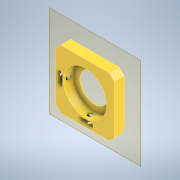
# Autodesk Inventor part: 20_Cube_Insert_Kinematic_KES400AMount_45_UPD_v3
Saved by Autodesk Inventor 2022 (Build 260153000, 153)
## iProperties
Created: 2021-11-15
Part Number: 20_Cube_Insert_Kinematic_KES400AMount_45_UPD_v3
Material: Generic
Document SubType Name: Modeling
Designer: diederichbenedict
Density: 1 g/cm^3
Appearance: Glossy - Gold
Author: diederichbenedict
Autodesk Inventor part; units mm, degrees
ref_plane "YZ Plane" through (0, 0, 0) normal (1, 0, 0) x (0, 1, 0)
ref_plane "XZ Plane" through (0, 0, 0) normal (0, 1, 0) x (-1, 0, 0)
ref_plane "XY Plane" through (0, 0, 0) normal (0, 0, 1) x (1, 0, 0)
ref_plane "Work Plane1" through (0, 0, 2) normal (0, 0, 1) x (1, 0, 0)
sketch "Sketch1" plane through (0, 0, 2) normal (0, 0, 1) x (1, 0, 0)
  circle A0 centre (-37.0712, 14) radius 3.25 construction
  circle A1 centre (-9.0712, -14) radius 3.25 construction
  line L0 (-21.8762, -24.9) -> (-21.8762, -17.08) construction
  line L1 (-21.8762, -17.08) -> (-20.0712, -17.08) construction
  arc A2 (-20.0712, -17.08) -> (-20.0712, -14.08) centre (-20.0712, -15.58) ccw construction
  line L2 (-20.0712, -14.08) -> (-21.8762, -14.08) construction
  line L3 (-21.8762, -14.08) -> (-21.8762, -3.0223) construction
  arc A3 (-21.8762, -3.0223) -> (-25.9925, 1.4242) centre (-23.0712, 0) ccw construction
  line L4 (-25.9925, 1.4242) -> (-37.0712, 1.4242) construction
  line L5 (-37.0712, 1.4242) -> (-37.0712, 3) construction
  arc A4 (-37.0712, 3) -> (-40.0712, 3) centre (-38.5712, 3) ccw construction
  line L6 (-40.0712, 3) -> (-40.0712, 1.4242) construction
  line L7 (-40.0712, 1.4242) -> (-47.9712, 1.4242) construction
  line L8 (-47.9712, 1.4242) -> (-47.9712, 17) construction
  line L9 (-47.9712, 17) -> (-44.3964, 17) construction
  line L10 (-44.3964, 17) -> (-40.0712, 21.3252) construction
  line L11 (-40.0712, 21.3252) -> (-40.0712, 24.9) construction
  line L12 (-40.0712, 24.9) -> (-6.0712, 24.9) construction
  line L13 (-6.0712, 24.9) -> (-6.0712, 21.3252) construction
  line L14 (-6.0712, 21.3252) -> (-1.746, 17) construction
  line L15 (-1.746, 17) -> (1.8288, 17) construction
  line L16 (1.8288, 17) -> (1.8288, -17) construction
  line L17 (1.8288, -17) -> (-1.746, -17) construction
  line L18 (-1.746, -17) -> (-6.1126, -21.3666) construction
  line L19 (-6.1126, -21.3666) -> (-6.1126, -24.9) construction
  line L20 (-6.1126, -24.9) -> (-21.8762, -24.9) construction
  circle A5 centre (-37.0712, -14) radius 3.25 construction
  circle A6 centre (-23.0712, 0) radius 12.45 construction
  circle A7 centre (-23.0712, 0) radius 12.7 construction
  line L21 (-37.0712, 14) -> (-9.0712, 14) construction
  line L22 (-9.0712, 14) -> (-9.0712, -14) construction
  line L23 (-9.0712, -14) -> (-37.0712, -14) construction
  line L24 (-37.0712, -14) -> (-37.0712, 14) construction
  line L25 (-5.5712, -17.5) -> (-5.5712, 17.5)
  line L26 (-5.5712, 17.5) -> (-40.5712, 17.5)
  line L27 (-40.5712, 17.5) -> (-40.5712, -17.5)
  line L28 (-40.5712, -17.5) -> (-5.5712, -17.5)
  circle A8 centre (-23.0712, 0) radius 12.8
  point P0 (0, 0)
  dimension "d0" = 3.5
  dimension "d1" = 0.1
  constraints: 16 end point, 4 parallel, 2 perpendicular, 1 centre point, 1 horizontal, 3 other
  measures "d0" distance between parallel lines of L22 L25
  measures "d1" radial gap between concentric circles of A7 A8
extrude "Extrusion1" add sketch "Sketch1" along normal blind 6
sketch "Sketch2" plane through (0, 0, 2) normal (0, 0, -1) x (-1, 0, 0)
  circle A0 centre (23.0712, 0) radius 12.8 projected
  circle A1 centre (23.0712, 0) radius 8.5824
  line L0 (5.5712, -17.5) -> (5.5712, 17.5) projected
  line L1 (5.5712, 17.5) -> (40.5712, 17.5) projected
  point P0 (0, 0)
  point P1 (5.5712, 0)
  point P2 (23.0712, 17.5)
  point P3 (5.5712, 0)
  point P4 (5.5712, 0)
  point P5 (5.5712, 0)
  point P6 (23.0712, 17.5)
  point P7 (23.0712, 17.5)
  point P8 (23.0712, 17.5)
  constraints: 8 midpoint, 3 vertical alignment, 2 coincident, 2 horizontal alignment, 1 centre point
extrude "Extrusion2" add sketch "Sketch2" against normal blind 0.5
sketch "Sketch3" plane through (0, 0, 2) normal (0, 0, -1) x (-1, 0, 0)
  circle A0 centre (9.0712, -14) radius 1.45 construction
  circle A1 centre (9.0712, -14) radius 2.45
  circle A2 centre (37.0712, -14) radius 1.45 projected
  circle A3 centre (37.0712, -14) radius 1.95
  point P0 (0, 0)
  dimension "d8" = 1
  dimension "d10" = 0.5
  constraints: 2 centre point
  measures "d8" radial gap between concentric circles of A0 A1
  measures "d10" radial gap between concentric circles of A2 A3
sketch "Sketch5" plane through (0, 0, 2) normal (0, 0, -1) x (-1, 0, 0)
  arc A0 (20.0712, -14.08) -> (20.0712, -17.08) centre (20.0712, -15.58) ccw projected
  arc A1 (26.0712, -17.08) -> (26.0712, -14.08) centre (26.0712, -15.58) ccw projected
  line L0 (37.0712, 3) -> (37.0712, -3) projected
  arc A2 (37.0712, -3) -> (40.0712, -3) centre (38.5712, -3) ccw projected
  line L1 (40.0712, -3) -> (40.0712, 3) projected
  arc A3 (40.0712, 3) -> (37.0712, 3) centre (38.5712, 3) ccw projected
  line L2 (26.0712, -14.08) -> (20.0712, -14.08) projected
  arc A4 (20.0712, -14.08) -> (20.0712, -17.08) centre (20.0712, -15.58) ccw projected
  line L3 (20.0712, -17.08) -> (26.0712, -17.08) projected
  arc A5 (26.0712, -17.08) -> (26.0712, -14.08) centre (26.0712, -15.58) ccw projected
  circle A6 centre (37.0712, -14) radius 1.45 projected
  circle A7 centre (23.0712, 0) radius 1.45 projected
  circle A8 centre (9.0712, -14) radius 1.45 projected
  circle A9 centre (37.0712, 14) radius 1.45 projected
  line L4 (-1.8288, -17) -> (-1.8288, 17) projected
  line L5 (-1.8288, 17) -> (1.746, 17) projected
  line L6 (1.746, 17) -> (6.0712, 21.3252) projected
  line L7 (6.0712, 21.3252) -> (6.0712, 24.9) projected
  line L8 (6.0712, 24.9) -> (40.0712, 24.9) projected
  line L9 (40.0712, 24.9) -> (40.0712, 21.3252) projected
  line L10 (40.0712, 21.3252) -> (44.3964, 17) projected
  line L11 (44.3964, 17) -> (47.9712, 17) projected
  line L12 (47.9712, 17) -> (47.9712, -17) projected
  line L13 (44.3964, -17) -> (47.9712, -17) projected
  line L14 (40.0712, -21.3252) -> (44.3964, -17) projected
  line L15 (40.0712, -24.9) -> (40.0712, -21.3252) projected
  line L16 (6.1126, -24.9) -> (40.0712, -24.9) projected
  line L17 (6.1126, -24.9) -> (6.1126, -21.3666) projected
  line L18 (6.1126, -21.3666) -> (1.746, -17) projected
  line L19 (1.746, -17) -> (-1.8288, -17) projected
  line L20 (40.5712, -17.5) -> (5.5712, -17.5) projected
  arc A10 (19.7251, -13.5) -> (18.2262, -15.0577) centre (19.7251, -15) ccw
  arc A11 (25.7274, -16.5) -> (25.7274, -16.5) centre (25.7274, -15) ccw
  line L21 (25.7274, -13.5) -> (25.7274, -13.5)
  arc A12 (19.7251, -13.5) -> (18.2262, -15.0577) centre (19.7251, -15) ccw
  line L22 (19.7251, -16.5) -> (19.7251, -16.5)
  arc A13 (25.7274, -16.5) -> (25.7274, -16.5) centre (25.7274, -15) ccw
  arc A14 (18.3936, -15.6908) -> (19.7251, -16.5) centre (19.7251, -15) ccw
  arc A15 (18.2262, -15.0577) -> (18.3936, -15.6908) centre (19.7251, -15) ccw
  arc A16 (18.3936, -15.6908) -> (19.7251, -16.5) centre (19.7251, -15) ccw
  arc A17 (18.2262, -15.0577) -> (18.3936, -15.6908) centre (19.7251, -15) ccw
  arc A18 (26.9396, -15.8835) -> (27.2262, -15.0582) centre (25.7274, -15) ccw
  arc A19 (26.9396, -15.8835) -> (27.2262, -15.0582) centre (25.7274, -15) ccw
  arc A20 (27.2262, -15.0582) -> (25.7274, -13.5) centre (25.7274, -15) ccw
  arc A21 (27.2262, -15.0582) -> (25.7274, -13.5) centre (25.7274, -15) ccw
  line L23 (19.7251, -16.5) -> (25.7274, -16.5)
  line L24 (25.7274, -13.5) -> (19.7251, -13.5)
  line L25 (19.7251, -13.5) -> (19.7251, -13.5)
  arc A22 (25.7274, -16.5) -> (26.9396, -15.8835) centre (25.7274, -15) ccw
  arc A23 (25.7274, -16.5) -> (26.9396, -15.8835) centre (25.7274, -15) ccw
  point P0 (0, 0)
  point P1 (40.0712, -3)
  point P2 (22.6287, -9.823)
  point P3 (22.6523, -12.823)
  point P4 (19.7251, -16.5)
  point P5 (25.7274, -16.5)
  point P6 (25.7274, -13.5)
  point P7 (19.7251, -13.5)
  dimension "d50" = 9
  dimension "d52" = 3
  dimension "d53" = 1.5
  dimension "d56" = 1.5
  dimension "d57" = 1.5
  dimension "d58" = 1.5
  dimension "d59" = 1
  constraints: 31 point on circle, 14 centre point, 10 end point, 7 parallel, 1 horizontal, 1 horizontal alignment, 1 point on line
  measures "d50" distance of A18.end A10.end
  measures "d52" distance between parallel lines of L22 L21
  measures "d53" radius of A20
  measures "d56" radius of A10
  measures "d57" radius of A14
  measures "d58" radius of A15
  measures "d59" distance between parallel lines of L20 L23
extrude "Extrusion5" cut sketch "Sketch5" against normal blind 8 contours L2 A11 L23 A14 A0 | A0 A14 A15 A10 L24 A11 L2 | A11 A1 L2 | L2 A1 A11
sketch "Sketch6" plane through (-40.5712, -17.5, 8) normal (0, -1, 0) x (1, 0, 0)
  line L0 (0, -6) -> (35, -6) projected
  line L1 (35, -6) -> (35, 0) projected
  line L2 (0, 0) -> (35, 0) projected
  line L3 (0, -6) -> (0, 0) projected
  line L4 (30.3, 0) -> (30.3, 0) projected
  circle A0 centre (17.5, -3) radius 1.45
  point P0 (40.5712, -8)
  point P1 (17.5, 0)
  point P2 (35, -3)
  dimension "d34" = 2.9
  constraints: 2 midpoint, 1 centre point, 1 horizontal alignment, 1 vertical alignment, 1 other
  measures "d34" diameter of A0
extrude "Extrusion6" cut sketch "Sketch6" against normal blind 8 contours A0
pattern_circular "Circular Pattern1" count 2 over 90 about axis through (-23.0712, 0, 2) along (0, 0, -1) of "Extrusion6"
chamfer "Chamfer1" distance 3 angle 45 4 edges at (-40.5712, 17.5, 5) (-5.5712, 17.5, 5) (-5.5712, -17.5, 5) (-40.5712, -17.5, 5)
hole "Hole1" at (-37.0712, -14, 2) direction (0, 0, 1) diameter 4 depth 0.1 tip angle 115
sketch "Sketch4" plane through (-5.5712, -17.5, 2) normal (1, 0, 0) x (0, 0, -1)
  line L0 (2, 4.45) -> (6, 4.45)
  line L1 (2, 1.55) -> (6, 1.55)
  line L2 (0, 0) -> (0, 35) projected
  arc A0 (2, 19) -> (2, 19) centre (1.5, 4.4206) ccw projected
  line L3 (-1.3741, 3.5) -> (-0.1, 5.5) projected
  line L4 (-1.3741, 3.5) -> (-0.1, 1.5) projected
  line L5 (-0.1, 5.5) -> (0.6045, 5.5)
  line L6 (0.6045, 5.5) -> (0.6045, 1.5)
  line L7 (0.6045, 1.5) -> (-0.1, 1.5)
  line L8 (-0.1, 1.5) -> (-0.1, 5.5)
  point P0 (2, 17.5)
  point P1 (-0.1, 1.5)
  constraints: 12 end point, 3 horizontal, 2 parallel, 1 perpendicular, 4 other
extrude "Extrusion4" cut sketch "Sketch4" against normal blind 8 contours L7 L8 L5 L2 | L2 L5 L6 L7 | L4 L3 L8
pattern_circular "Circular Pattern2" count 2 over 90 about axis through (-23.0712, 0, 2) along (0, 0, -1) of "Extrusion5"
equation "\"d50\" = d49"
equation "\"d52\" = d51"
equation "\"d53\" = d55"
equation "\"d56\" = d55"
equation "\"d49\" = 9"
equation "\"d51\" = 3"
equation "\"d55\" = 1.5"
body "Solid1"
